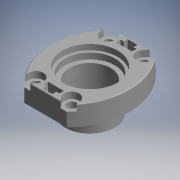
# Autodesk Inventor part: Abdeckkappe_LZ80
Saved by Autodesk Inventor 2017.3 (Build 213256000, 256)
## iProperties
Part Number: Abdeckkappe_LZ80
Material: Generic
Catalog Web Link: www.cadenas.de
Description: LZ80 Abdeckkappe-Bauteil LZ80
Vendor: ROSEKRIEGER
Document SubType Name: Modeling
Designer: partserver
Manufacturer: ROSEKRIEGER
Mass: 81.7882 g
Surface Area: 274.945 cm^2
Volume: 81.7882 cm^3
Density: 1 g/cm^3
Appearance: PSOLRGB-192-192-192
Category: PARTsolutions
Company: ROSEKRIEGER
Title: Abdeckkappe_LZ80
Author: Cadenas PARTsolutions
Comments: Bauteil LZ80
PSOL_IDENT_0: {$CADENAS_DATA\23d-libs\rose_krieger\linearkomponenten\pool_lineartechnik\_hubsaeule_zyliinder\elekt
PSOL_IDENT_1: rozylinder\elekzyl_lz80\lz80_abdeckkappe.prj},173 {VTYP=3D},{NB=Abdeckkappe_LZ80},{LINA=Abdeckkappe_
PSOL_IDENT_2: LZ80},{NN=LZ80 Abdeckkappe},{DATE=02.12.2020 11:16:41},{GEOMDATE=12.12.2006},{VERSION=},{LINEID=10},
PSOL_IDENT_3: {WBVAR=},{WBNUMERIC=}  {NB=Abdeckkappe_LZ80},{LINA=Abdeckkappe_LZ80},{KT=DUMMY},{IDNR=},{ARTIKEL=Abd
PSOL_IDENT_4: eckkappe_LZ80},{BREITE=90.000},{HOEKAP=20.000},{XRADKONTUR=25.250},{RADKONTUR=64.890},{GESHOE=41.000
PSOL_IDENT_5: },{ZENTA=56.000},{ZENTB=50.500},{TIEFZENTB=6.000},{TIEFZENTA=5.500},{DURCHA=50.000},{ZENTC=44.000},{
PSOL_IDENT_6: TIEFZENTC=20.000},{RADIUS2=0.500},{RADIUS3=1.000},{DURCHB=41.500},{NUTBR1=16.000},{NUTBR2=10.000},{N
PSOL_IDENT_7: UTTIEFE1=8.500},{NUTTIEFE2=4.500},{NUTAB=2.000},{SENKDURCHB=9.000},{ABSENKLAE=73.000},{ABSENKBR=36.0
PSOL_IDENT_8: 00},{SENKDURCHT=6.400},{SENKDURCHK=15.000},{WINKPUNKT=15.300},{WINKPUNKT2=26.000},{ABEBENE=5.500}
NB: Abdeckkappe_LZ80
NN: LZ80 Abdeckkappe
NT: Bauteil LZ80
NBSYN: $ARTIKEL.
LINA: Abdeckkappe_LZ80
CATALOG: RK Rose+Krieger
ARTIKEL: Abdeckkappe_LZ80
BREITE: 90
HOEKAP: 20
XRADKONTUR: 25.25
RADKONTUR: 64.89
GESHOE: 41
ZENTA: 56
ZENTB: 50.5
TIEFZENTB: 6
TIEFZENTA: 5.5
DURCHA: 50
ZENTC: 44
TIEFZENTC: 20
RADIUS2: 0.5
RADIUS3: 1
DURCHB: 41.5
NUTBR1: 16
NUTBR2: 10
NUTTIEFE1: 8.5
NUTTIEFE2: 4.5
NUTAB: 2
SENKDURCHB: 9
ABSENKLAE: 73
ABSENKBR: 36
SENKDURCHT: 6.4
SENKDURCHK: 15
WINKPUNKT: 15.3
WINKPUNKT2: 26
ABEBENE: 5.5
SUPPLIER: ROSEKRIEGER
ARTICLENO: Abdeckkappe_LZ80
BOMINFO: Abdeckkappe_LZ80
CREATOR: CADENAS GmbH
Autodesk Inventor part; units mm, degrees
ref_plane "YZ Plane" through (0, 0, 0) normal (1, 0, 0) x (0, 1, 0)
ref_plane "XZ Plane" through (0, 0, 0) normal (0, 1, 0) x (-1, 0, 0)
ref_plane "XY Plane" through (0, 0, 0) normal (0, 0, 1) x (1, 0, 0)
sketch "Skizze_1" plane through (0, 0, 0) normal (0, 0, 1) x (1, 0, 0)
  arc A0 (-21.5016, 45) -> (-21.5016, -45) centre (25.25, 0) ccw
  line L0 (-21.5016, -45) -> (21.5016, -45)
  arc A1 (21.5016, -45) -> (21.5016, 45) centre (-25.25, 0) ccw
  line L1 (21.5016, 45) -> (-21.5016, 45)
  constraints: 4 end point, 4 point on circle, 2 centre point
extrude "Extrusion1" add sketch "Skizze_1" along normal blind 20
sketch "Skizze_2" plane through (0, 0, 0) normal (0, 1, 0) x (-1, 0, 0)
  line L0 (-25.25, -50) -> (-25.25, 50)
  line L1 (40.14, -0.5) -> (40.14, 1)
  line L2 (40.14, 1) -> (39.64, 1)
  arc A0 (38.64, 0) -> (39.64, 1) centre (38.64, 1) ccw
  line L3 (38.64, 0) -> (38.64, -0.5)
  line L4 (38.64, -0.5) -> (40.14, -0.5)
  constraints: 10 end point, 2 point on circle, 1 centre point
revolve "Revolution1" cut sketch "Skizze_2" angle 360 about axis through (25.25, 0, -50) along (0, 0, -1)
sketch "Skizze_3" plane through (0, 0, 0) normal (0, 1, 0) x (-1, 0, 0)
  line L0 (25.25, 50) -> (25.25, -50)
  arc A0 (-39.64, 1) -> (-38.64, 0) centre (-38.64, 1) ccw
  line L1 (-39.64, 1) -> (-40.14, 1)
  line L2 (-40.14, 1) -> (-40.14, -0.5)
  line L3 (-40.14, -0.5) -> (-38.64, -0.5)
  line L4 (-38.64, -0.5) -> (-38.64, 0)
  constraints: 10 end point, 2 point on circle, 1 centre point
revolve "Revolution2" cut sketch "Skizze_3" angle 360 about axis through (-25.25, 0, 50) along (0, 0, 1)
sketch "Skizze_4" plane through (0, 0, 0) normal (1, 0, 0) x (0, 1, 0)
  arc A0 (44, 0) -> (45, 1) centre (44, 1) ccw
  line L0 (44, 0) -> (45, 0)
  line L1 (45, 0) -> (45, 1)
  constraints: 4 end point, 2 point on circle, 1 centre point
extrude "Extrusion2" cut sketch "Skizze_4" along normal mid plane 90
sketch "Skizze_5" plane through (0, 0, 0) normal (1, 0, 0) x (0, 1, 0)
  line L0 (-45, 1) -> (-45, 0)
  line L1 (-45, 0) -> (-44, 0)
  arc A0 (-45, 1) -> (-44, 0) centre (-44, 1) ccw
  constraints: 4 end point, 2 point on circle, 1 centre point
extrude "Extrusion3" cut sketch "Skizze_5" along normal mid plane 90
sketch "Skizze_6" plane through (0, 0, 0) normal (0, 0, 1) x (1, 0, 0)
  circle A0 centre (0, 0) radius 25
  constraints: 1 centre point
extrude "Extrusion4" add sketch "Skizze_6" along normal blind 41
sketch "Skizze_7" plane through (0, 0, 0) normal (0, 1, 0) x (-1, 0, 0)
  line L0 (0, 41) -> (0, 0)
  line L1 (0, 0) -> (-28, 0)
  line L2 (-28, 0) -> (-28, 5.5)
  line L3 (-28, 5.5) -> (-25.25, 5.5)
  line L4 (-25.25, 5.5) -> (-25.25, 11.5)
  line L5 (-25.25, 11.5) -> (-20.75, 11.5)
  line L6 (-20.75, 11.5) -> (-20.75, 21)
  line L7 (-20.75, 21) -> (-22, 21)
  line L8 (-22, 21) -> (-22, 41)
  line L9 (-22, 41) -> (0, 41)
  line L10 (0, 41) -> (0, 0)
  constraints: 22 end point
revolve "Revolution3" cut sketch "Skizze_7" angle 360 about axis through (0, 0, 41) along (0, 0, 1)
sketch "Skizze_8" plane through (0, 0, 0) normal (0, 0, 1) x (1, 0, 0)
  line L0 (-8, 39) -> (-8, 34.5)
  line L1 (-8, 34.5) -> (8, 34.5)
  line L2 (8, 34.5) -> (8, 39)
  line L3 (8, 39) -> (5, 39)
  line L4 (5, 39) -> (5, 43)
  line L5 (5, 43) -> (-5, 43)
  line L6 (-5, 43) -> (-5, 39)
  line L7 (-5, 39) -> (-8, 39)
  constraints: 16 end point
extrude "Extrusion5" cut sketch "Skizze_8" along normal blind 20
sketch "Skizze_9" plane through (0, 0, 0) normal (0, 0, 1) x (1, 0, 0)
  line L0 (-8, -34.5) -> (-8, -39)
  line L1 (-8, -39) -> (-5, -39)
  line L2 (-5, -39) -> (-5, -43)
  line L3 (-5, -43) -> (5, -43)
  line L4 (5, -43) -> (5, -39)
  line L5 (5, -39) -> (8, -39)
  line L6 (8, -39) -> (8, -34.5)
  line L7 (8, -34.5) -> (-8, -34.5)
  constraints: 16 end point
extrude "Extrusion6" cut sketch "Skizze_9" along normal blind 20
sketch "Skizze_10" plane through (0, 0, 6.4) normal (0, 0, 1) x (1, 0, 0)
  circle A0 centre (18, 36.5) radius 4.5
  constraints: 1 centre point
extrude "Extrusion7" cut sketch "Skizze_10" along normal mid plane 40
pattern_linear "Rectangular Pattern1" count 2 spacing 36 along (-1, 0, 0) count 2 spacing 73 along (0, -1, 0) of "Extrusion7"
sketch "Skizze_12" plane through (0, 0, 6.4) normal (0, 0, 1) x (1, 0, 0)
  arc A0 (12.2226, 41.2825) -> (25.4357, 35.5199) centre (18, 36.5) ccw
  line L0 (25.4357, 35.5199) -> (26, 39.8014)
  arc A1 (26, 39.8014) -> (21.5016, 45) centre (-25.25, 0) ccw
  line L1 (21.5016, 45) -> (15.3, 45)
  line L2 (15.3, 45) -> (12.2226, 41.2825)
  constraints: 6 end point, 4 point on circle, 2 centre point
extrude "Extrusion8" cut sketch "Skizze_12" against normal blind 6.4
sketch "Skizze_13" plane through (0, 0, 6.4) normal (0, 0, 1) x (1, 0, 0)
  line L0 (-26, 39.8014) -> (-25.4357, 35.5199)
  arc A0 (-25.4357, 35.5199) -> (-12.2226, 41.2825) centre (-18, 36.5) ccw
  line L1 (-12.2226, 41.2825) -> (-15.3, 45)
  line L2 (-15.3, 45) -> (-21.5016, 45)
  arc A1 (-21.5016, 45) -> (-26, 39.8014) centre (25.25, 0) ccw
  constraints: 6 end point, 4 point on circle, 2 centre point
extrude "Extrusion9" cut sketch "Skizze_13" against normal blind 6.4
sketch "Skizze_14" plane through (0, 0, 6.4) normal (0, 0, 1) x (1, 0, 0)
  arc A0 (25.4357, -35.5199) -> (12.2226, -41.2825) centre (18, -36.5) ccw
  line L0 (12.2226, -41.2825) -> (15.3, -45)
  line L1 (15.3, -45) -> (21.5016, -45)
  arc A1 (21.5016, -45) -> (26, -39.8014) centre (-25.25, 0) ccw
  line L2 (26, -39.8014) -> (25.4357, -35.5199)
  constraints: 6 end point, 4 point on circle, 2 centre point
extrude "Extrusion10" cut sketch "Skizze_14" against normal blind 6.4
sketch "Skizze_15" plane through (0, 0, 6.4) normal (0, 0, 1) x (1, 0, 0)
  arc A0 (-26, -39.8014) -> (-21.5016, -45) centre (25.25, 0) ccw
  line L0 (-21.5016, -45) -> (-15.3, -45)
  line L1 (-15.3, -45) -> (-12.2226, -41.2825)
  arc A1 (-12.2226, -41.2825) -> (-25.4357, -35.5199) centre (-18, -36.5) ccw
  line L2 (-25.4357, -35.5199) -> (-26, -39.8014)
  constraints: 6 end point, 4 point on circle, 2 centre point
extrude "Extrusion11" cut sketch "Skizze_15" against normal blind 6.4
ref_plane "EPANDOPPRO_XY" through (0, 0, 20) normal (0, 0, 1) x (1, 0, 0)
ref_plane "EPANDOPPRO_YZ" through (0, 0, 20) normal (1, 0, 0) x (0, 1, 0)
ref_plane "EPANDOPPRO_ZX" through (0, 0, 20) normal (0, 1, 0) x (0, 0, 1)
ref_plane "EPDICHTR_XY" through (0, 0, 5.5) normal (0, 0, 1) x (1, 0, 0)
ref_plane "EPDICHTR_YZ" through (0, 0, 5.5) normal (1, 0, 0) x (0, 1, 0)
ref_plane "EPDICHTR_ZX" through (0, 0, 5.5) normal (0, 1, 0) x (0, 0, 1)
ref_plane "EPZYL_XY" through (18, 36.5, 6.4) normal (0, 0, 1) x (1, 0, 0)
ref_plane "EPZYL_YZ" through (18, 36.5, 6.4) normal (1, 0, 0) x (0, 1, 0)
ref_plane "EPZYL_ZX" through (18, 36.5, 6.4) normal (0, 1, 0) x (0, 0, 1)
ref_plane "EPZYL2_XY" through (-18, 36.5, 6.4) normal (0, 0, 1) x (1, 0, 0)
ref_plane "EPZYL2_YZ" through (-18, 36.5, 6.4) normal (1, 0, 0) x (0, 1, 0)
ref_plane "EPZYL2_ZX" through (-18, 36.5, 6.4) normal (0, 1, 0) x (0, 0, 1)
ref_plane "EPZYL3_XY" through (-18, -36.5, 6.4) normal (0, 0, 1) x (1, 0, 0)
ref_plane "EPZYL3_YZ" through (-18, -36.5, 6.4) normal (1, 0, 0) x (0, 1, 0)
ref_plane "EPZYL3_ZX" through (-18, -36.5, 6.4) normal (0, 1, 0) x (0, 0, 1)
ref_plane "EPZYL4_XY" through (18, -36.5, 6.4) normal (0, 0, 1) x (1, 0, 0)
ref_plane "EPZYL4_YZ" through (18, -36.5, 6.4) normal (1, 0, 0) x (0, 1, 0)
ref_plane "EPZYL4_ZX" through (18, -36.5, 6.4) normal (0, 1, 0) x (0, 0, 1)
body "Solid1"
